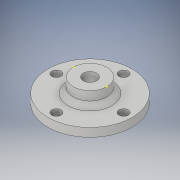
# Autodesk Inventor part: FlywheelMount
Saved by Autodesk Inventor 2018 (Build 220112000, 112)
## iProperties
Created: 2019-06-24
Part Number: FlywheelMount
Material: Generic
Document SubType Name: Modeling
Designer: anirudh
Density: 1 g/cm^3
Appearance: Default
Author: anirudh
Autodesk Inventor part; units mm, degrees
ref_plane "YZ Plane" through (0, 0, 0) normal (1, 0, 0) x (0, 1, 0)
ref_plane "XZ Plane" through (0, 0, 0) normal (0, 1, 0) x (-1, 0, 0)
ref_plane "XY Plane" through (0, 0, 0) normal (0, 0, 1) x (1, 0, 0)
sketch "Sketch1" plane through (0, 0, 0) normal (0, 1, 0) x (-1, 0, 0)
  circle A0 centre (0, 0) radius 15.875
  circle A1 centre (0, 0) radius 6.35
  circle A2 centre (0, 12.7) radius 1.75
  circle A3 centre (-12.7, 0) radius 1.75
  circle A4 centre (0, -12.7) radius 1.75
  circle A5 centre (12.7, 0) radius 1.75
  dimension "d1" = 12.7
  dimension "d6" = 3.5
  dimension "d7" = 3.5
  dimension "d8" = 3.5
  dimension "d9" = 3.5
  constraints: 6 centre point, 2 coincident
  measures "d1" diameter of A1
  measures "d6" diameter of A2
  measures "d7" diameter of A3
  measures "d8" diameter of A4
  measures "d9" diameter of A5
extrude "Extrusion1" add sketch "Sketch1" along normal blind 3.2258
sketch "Sketch2" plane through (0, 3.2258, 0) normal (0, 1, 0) x (1, 0, 0)
  circle A0 centre (0, 0) radius 6.35
  circle A1 centre (0, 0) radius 2.54
  dimension "d12" = 5.08
  constraints: 2 centre point, 2 coincident
  measures "d12" diameter of A1
extrude "Extrusion2" add sketch "Sketch2" along normal blind 5.3086
sketch "Sketch3" plane through (0, 8.5344, 0) normal (0, 1, 0) x (1, 0, 0)
  line L0 (0, 0) -> (6.35, 0)
  circle A0 centre (0, 0) radius 6.35 projected
  line L1 (0, 0) -> (-6.35, 0)
  constraints: 4 end point, 2 horizontal, 2 point on circle
ref_plane "Work Plane3" through (0, 8.5344, 0) normal (1, 0, 0) x (0, 1, 0)
sketch "Sketch5" plane through (0, 3.2258, 0) normal (0, 1, 0) x (1, 0, 0)
  circle A0 centre (0, 0) radius 6.35
  circle A1 centre (0, 0) radius 8.255
  dimension "d17" = 16.51
  constraints: 2 centre point, 2 coincident
  measures "d17" diameter of A1
extrude "Extrusion3" add sketch "Sketch5" along normal blind 1.905
chamfer "Chamfer1" distance 1.905 angle 45 1 edges at (-8.255, 5.1308, 0)
chamfer "Chamfer2" distance 0.635 angle 45 1 edges at (6.35, 3.2258, 0)
body "Solid1"
